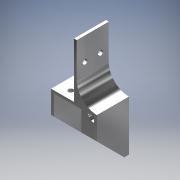
# Autodesk Inventor part: Pneumatic Connector
Saved by Autodesk Inventor 2019.4 (Build 234330000, 330)
## iProperties
Created: 2020-01-11
Part Number: Pneumatic Connector
Material: Aluminum 6061
Document SubType Name: Modeling
Designer: Mark
Mass: 91.5208 g
Surface Area: 184.578 cm^2
Volume: 33.8966 cm^3
Density: 2.7 g/cm^3
Appearance: Aluminum - Flat
Author: Mark
Autodesk Inventor part; units mm, degrees
ref_plane "YZ Plane" through (0, 0, 0) normal (1, 0, 0) x (0, 1, 0)
ref_plane "XZ Plane" through (0, 0, 0) normal (0, 1, 0) x (-1, 0, 0)
ref_plane "XY Plane" through (0, 0, 0) normal (0, 0, 1) x (1, 0, 0)
sketch "Sketch1" plane through (0, 0, 0) normal (0, 0, 1) x (1, 0, 0)
  line L0 (-25, -25) -> (25, -25)
  line L1 (25, -25) -> (25, 25)
  line L2 (25, 25) -> (-25, 25)
  line L3 (-25, 25) -> (-25, -25)
  line L4 (-25, -25) -> (25, 25) construction
  line L5 (25, -25) -> (-25, 25) construction
  line L6 (-25, 25) -> (25, 25)
  line L7 (25, 25) -> (25, 30)
  line L8 (25, 30) -> (-25, 30)
  line L9 (-25, 30) -> (-25, 25)
  circle A0 centre (-8.5, -2.5) radius 6.5
  point P0 (0, 0)
  dimension "d1" = 50
  dimension "d2" = 50
  dimension "d3" = 5
  dimension "d16" = 25
  dimension "d17" = 25
  dimension "d18" = 13
  dimension "d20" = 22.5
  dimension "d21" = 50
  dimension "d22" = 16.5
  constraints: 20 end point, 4 parallel, 2 horizontal, 2 perpendicular, 1 centre point
  measures "d1" distance of L2.end L1.end
  measures "d2" distance of L1.end L0.end
  measures "d3" distance of L7.end L6.end
  measures "d16" distance from line of point (0, 0) L0
  measures "d17" distance from line of point (0, 0) L3
  measures "d18" diameter of A0
  measures "d20" distance from line of L0 A0.centre
  measures "d21" distance of L7.end L8.end
  measures "d22" distance from line of L3 A0.centre
extrude "Extrusion1" add sketch "Sketch1" along normal blind 5
sketch "Sketch2" plane through (0, 0, 5) normal (0, 0, 1) x (1, 0, 0)
  line L0 (25, 30) -> (-25, 30) projected
  line L1 (-25, 30) -> (25, 30)
  line L2 (25, 30) -> (25, 27)
  line L3 (25, 27) -> (-25, 27)
  line L4 (-25, 27) -> (-25, 30)
  line L5 (-25, 27) -> (-22, 27)
  line L6 (-22, 27) -> (-22, -25)
  line L7 (-22, -25) -> (-25, -25)
  line L8 (-25, -25) -> (-25, 27)
  line L9 (25, -25) -> (22, -25)
  line L10 (22, -25) -> (22, 27)
  line L11 (22, 27) -> (25, 27)
  line L12 (25, 27) -> (25, -25)
  line L13 (25, -25) -> (25, 30) projected
  point P0 (0, 0)
  dimension "d6" = 50
  dimension "d7" = 3
  dimension "d8" = 3
  dimension "d9" = 52
  dimension "d10" = 3
  constraints: 24 end point, 6 parallel, 3 horizontal, 3 perpendicular, 2 point on line, 1 collinear
  measures "d6" distance of L2.end L3.end
  measures "d7" distance of L1.end L2.end
  measures "d8" distance of L6.end L7.end
  measures "d9" distance of L5.end L6.end
  measures "d10" distance of L10.end L11.end
extrude "Extrusion2" add sketch "Sketch2" along normal blind 30
chamfer "Chamfer1" distance 30 angle 45 2 edges at (23.5, -25, 35) (-23.5, -25, 35)
sketch "Sketch3" plane through (-25, 30, 0) normal (0, 1, 0) x (1, 0, 0)
  line L0 (25, -35) -> (28, -35)
  line L1 (28, -35) -> (28, 0)
  line L2 (28, 0) -> (25, 0)
  line L3 (25, 0) -> (25, -35)
  line L4 (50, -35) -> (0, -35) projected
  line L5 (50, 0) -> (50, -35) projected
  dimension "d23" = 3
  dimension "d24" = 25
  constraints: 8 end point, 2 parallel, 1 collinear, 1 horizontal, 1 perpendicular
  measures "d23" distance of L2.end L1.end
  measures "d24" distance between parallel lines of L5 L3
extrude "Extrusion3" add sketch "Sketch3" along normal blind 60
fillet "Fillet1" radius 22 1 edges at (3, 30, 17.5)
sketch "Sketch4" plane through (-22, 27, 5) normal (0, -1, 0) x (1, 0, 0)
  circle A0 centre (9.5, 21) radius 2.75
  circle A1 centre (9.5, 7) radius 2.75
  line L0 (0, 0) -> (0, 30) projected
  line L1 (0, 30) -> (44, 30) projected
  line L2 (0, 0) -> (44, 0) projected
  point P0 (22, -5)
  dimension "d28" = 5.5
  dimension "d29" = 5.5
  dimension "d30" = 9.5
  dimension "d31" = 9.5
  dimension "d32" = 9
  dimension "d33" = 7
  constraints: 2 centre point
  measures "d28" diameter of A0
  measures "d29" diameter of A1
  measures "d30" distance from line of L0 A0.centre
  measures "d31" distance from line of A1.centre L0
  measures "d32" distance from line of L1 A0.centre
  measures "d33" distance from line of L2 A1.centre
extrude "Extrusion4" cut sketch "Sketch4" against normal blind 60
sketch "Sketch5" plane through (3, 90, 35) normal (1, 0, 0) x (0, 0, -1)
  circle A0 centre (9, -25) radius 2.75
  circle A1 centre (26, -25) radius 2.75
  line L0 (0, 0) -> (35, 0) projected
  line L1 (0, -38) -> (0, 0) projected
  line L2 (35, -38) -> (35, 0) projected
  point P0 (35, -90)
  dimension "d36" = 5.5
  dimension "d37" = 5.5
  dimension "d38" = 25
  dimension "d39" = 25
  dimension "d40" = 9
  dimension "d41" = 9
  constraints: 2 centre point
  measures "d36" diameter of A0
  measures "d37" diameter of A1
  measures "d38" distance from line of L0 A1.centre
  measures "d39" distance from line of L0 A0.centre
  measures "d40" distance from line of L1 A0.centre
  measures "d41" distance from line of L2 A1.centre
extrude "Extrusion5" cut sketch "Sketch5" against normal blind 60
body "Solid1"
